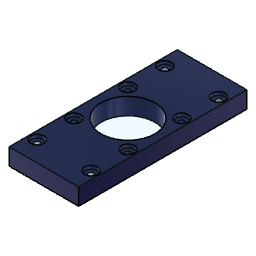
Braço Robótico 3.0(Tampa do motor da cerro do braço) v10 (Autodesk Fusion 360 design; units mm, degrees)
Autodesk Fusion 360 part; units mm, degrees
sketch "Sketch1" plane through (0, 0, 0) normal (0, 0, 1) x (1, 0, 0)
  line L0 (0, 0) -> (20.646, 0)
  line L1 (20.646, 0) -> (20.646, 50)
  line L2 (20.646, 50) -> (0, 50)
  line L3 (0, 50) -> (0, 0)
  dimension "d1" = 20.646
  dimension "d2" = 50
  constraint horizontal L0
  constraint vertical L1
  constraint horizontal L2
  constraint vertical L3
  constraint coincident L0.start L3.end
  measures "d1" distance of L0.start L0.end
  measures "d2" distance of L0.start L2.end
extrude "Extrude1" add sketch "Sketch1" along normal blind 5
sketch "Sketch2" plane through (0, 0, 5) normal (0, 0, 1) x (-1, 0, 0)
  line L0 (0, -50) -> (0, 0)
  line L1 (0, 0) -> (-20.646, 0)
  line L2 (-20.646, 0) -> (-20.646, -50)
  line L3 (-20.646, -50) -> (0, -50)
sketch "Sketch3" plane through (0, 0, 5) normal (0, 0, 1) x (-1, 0, 0)
  line L0 (-20.646, 0) -> (-20.646, -50)
  line L1 (0, -50) -> (0, 0)
  circle A0 centre (-10.323, -25) radius 8.0085
  dimension "d5" = 16.017
  measures "d5" diameter of A0
extrude "Extrude2" cut sketch "Sketch3" against normal blind 10
sketch "Sketch4" plane through (0, 0, 5) normal (0, 0, 1) x (-1, 0, 0)
  circle A0 centre (-10.323, -25) radius 8.0085
  line L0 (-10.323, -25) -> (-2.3221, -33.0009)
  line L1 (-10.323, -25) -> (-2.3221, -16.9991)
  line L2 (-10.323, -25) -> (-18.3239, -16.9991)
  line L3 (-10.323, -25) -> (-18.3239, -33.0009)
hole "Hole1" at (2.3221, 16.9991, 5) at (2.3221, 33.0009, 5) at (18.3239, 33.0009, 5) at (18.3239, 16.9991, 5) direction (0, 0, -1) diameter 1.623 depth 16 tip angle 180 counterbore diameter 3.9 counterbore depth 1
sketch "Sketch5" plane through (0, 0, 5) normal (0, 0, 1) x (-1, 0, 0)
  circle A0 centre (-2.3221, -33.0009) radius 1.95
  line L0 (-2.3221, -33.0009) -> (-2.3221, -44.0009)
  circle A1 centre (-18.3239, -33.0009) radius 1.95
  line L1 (-18.3239, -33.0009) -> (-18.3239, -44.0009)
  circle A2 centre (-2.3221, -16.9991) radius 1.95
  line L2 (-2.3221, -16.9991) -> (-2.3221, -5.9991)
  circle A3 centre (-18.3239, -16.9991) radius 1.95
  line L3 (-18.3239, -16.9991) -> (-18.3239, -5.9991)
  dimension "d16" = 11
  dimension "d17" = 11
  dimension "d18" = 11
  dimension "d19" = 11
  constraint coincident A0.centre L0.start
  constraint vertical L1
  constraint coincident A1.centre L1.start
  constraint parallel L0 L1
  constraint coincident A2.centre L2.start
  constraint coincident A3.centre L3.start
  constraint vertical L3
  measures "d16" distance of A0.centre L0.end
  measures "d17" distance of A1.centre L1.end
  measures "d18" distance of A2.centre L2.end
  measures "d19" distance of A3.centre L3.end
hole "Hole2" at (2.3221, 5.9991, 5) at (18.3239, 5.9991, 5) at (18.3239, 44.0009, 5) at (2.3221, 44.0009, 5) direction (0, 0, -1) diameter 1.623 end through all counterbore diameter 3.9 counterbore depth 1
thread "Thread1" "ISO Metric profile 2.0 M2x0.4 6H"
sketch "Sketch6" plane through (0, 0, 5) normal (0, 0, 1) x (-1, 0, 0)
